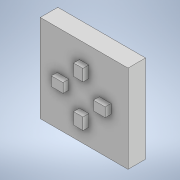
# Autodesk Inventor part: led-bracket
Saved by Autodesk Inventor 2021 (Build 250183000, 183)
## iProperties
Created: 2020-12-30
Part Number: led-bracket
Material: Generic
Document SubType Name: Modeling
Designer: Luke Kamols
Density: 1 g/cm^3
Appearance: Default
Author: Luke Kamols
Autodesk Inventor part; units mm, degrees
ref_plane "YZ Plane" through (0, 0, 0) normal (1, 0, 0) x (0, 1, 0)
ref_plane "XZ Plane" through (0, 0, 0) normal (0, 1, 0) x (-1, 0, 0)
ref_plane "XY Plane" through (0, 0, 0) normal (0, 0, 1) x (1, 0, 0)
sketch "Sketch1" plane through (0, 0, 0) normal (0, 0, 1) x (1, 0, 0)
  line L0 (0, 0) -> (15, 0)
  line L1 (15, 0) -> (15, 15)
  line L2 (15, 15) -> (0, 15)
  line L3 (0, 15) -> (0, 0)
  dimension "d0" = 15
  dimension "d1" = 15
  constraints: 8 end point, 2 parallel, 1 horizontal, 1 perpendicular
  measures "d0" distance of L2.end L1.end
  measures "d1" distance of L1.end L0.end
extrude "Extrusion1" add sketch "Sketch1" along normal blind 3
sketch "Sketch2" plane through (0, 0, 3) normal (0, 0, 1) x (1, 0, 0)
  line L0 (0, 0) -> (15, 0) projected
  line L1 (15, 0) -> (15, 15) projected
  line L2 (0, 0) -> (15, 15)
  line L3 (15, 15) -> (0, 15) projected
  line L4 (0, 15) -> (15, 0)
  line L5 (7.5, 7.5) -> (10.1, 7.5)
  line L6 (10.1, 7.5) -> (10.1, 8.3)
  line L7 (10.1, 8.3) -> (12.1, 8.3)
  line L8 (12.1, 8.3) -> (12.1, 6.7)
  line L9 (12.1, 6.7) -> (10.1, 6.7)
  line L10 (10.1, 6.7) -> (10.1, 7.5)
  line L11 (7.5, 7.5) -> (7.5, 4.9)
  line L12 (7.5, 4.9) -> (8.3, 4.9)
  line L13 (8.3, 4.9) -> (8.3, 2.9)
  line L14 (8.3, 2.9) -> (6.7, 2.9)
  line L15 (6.7, 2.9) -> (6.7, 4.9)
  line L16 (6.7, 4.9) -> (7.5, 4.9)
  line L17 (7.5, 7.5) -> (4.9, 7.5)
  line L18 (4.9, 7.5) -> (4.9, 6.7)
  line L19 (4.9, 6.7) -> (2.9, 6.7)
  line L20 (2.9, 6.7) -> (2.9, 8.3)
  line L21 (2.9, 8.3) -> (4.9, 8.3)
  line L22 (4.9, 8.3) -> (4.9, 7.5)
  line L23 (7.5, 7.5) -> (7.5, 10.1)
  line L24 (7.5, 10.1) -> (8.3, 10.1)
  line L25 (8.3, 10.1) -> (8.3, 12.1)
  line L26 (8.3, 12.1) -> (6.7, 12.1)
  line L27 (6.7, 12.1) -> (6.7, 10.1)
  line L28 (6.7, 10.1) -> (7.5, 10.1)
  dimension "d4" = 2.6
  dimension "d5" = 0.8
  dimension "d6" = 2
  dimension "d7" = 1.6
  dimension "d8" = 2.6
  dimension "d9" = 0.8
  dimension "d10" = 2
  dimension "d11" = 1.6
  dimension "d12" = 2.6
  dimension "d13" = 2
  dimension "d14" = 2.6
  dimension "d15" = 2
  constraints: 52 end point, 20 perpendicular, 4 point on line, 3 horizontal, 1 midpoint, 1 vertical
  measures "d4" distance of L5.start L5.end
  measures "d5" distance of L5.end L6.end
  measures "d6" distance of L6.end L7.end
  measures "d7" distance of L7.end L8.end
  measures "d8" distance of L5.start L11.end
  measures "d9" distance of L11.end L12.end
  measures "d10" distance of L12.end L13.end
  measures "d11" distance of L13.end L14.end
  measures "d12" distance of L5.start L17.end
  measures "d13" distance of L18.end L19.end
  measures "d14" distance of L5.start L23.end
  measures "d15" distance of L24.end L25.end
extrude "Extrusion2" add sketch "Sketch2" along normal blind 1 contours L12 L13 L14 L15 L16 | L18 L19 L20 L21 L22 | L6 L7 L8 L9 L10 | L28 L27 L26 L25 L24
body "Solid1"
